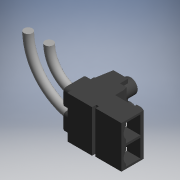
# Autodesk Inventor part: 4021832 2GD-1RR7.62-CLP-CBL
Saved by Autodesk Inventor 2017.3 (Build 213256000, 256)
## iProperties
Part Number: 4021832 2GD-1RR7.62-CLP-CBL
Material: Generic
Catalog Web Link: www.cadenas.de
Description: CMMT-plug-plug
Vendor: FESTO
Document SubType Name: Modeling
Designer: partserver
Manufacturer: FESTO
Mass: 2.92165 g
Surface Area: 28.4922 cm^2
Volume: 2.92165 cm^3
Density: 1 g/cm^3
Appearance: PSOLRGB-80-80-80
Category: PARTsolutions
Company: FESTO
Title: 4021832 2GD-1RR7.62-CLP-CBL
Author: Cadenas PARTsolutions
Comments: plug
PSOL_IDENT_0: {$CADENAS_DATA\23d-libs\festo\parts\c\cmmt\parts\cmmt_plug.prj},197 {VTYP=3D},{NB=4021832 2GD-1RR7.6
PSOL_IDENT_1: 2-CLP-CBL},{LINA=4021832 2GD-1RR7.62-CLP-CBL},{NN=CMMT-plug},{DATE=30.08.2019 14:28:39},{GEOMDATE=29
PSOL_IDENT_2: .03.2018 10:55:00},{VERSION=},{LINEID=10},{WBVAR=},{WBNUMERIC=}  {NB=4021832 2GD-1RR7.62-CLP-CBL},{L
PSOL_IDENT_3: INA=4021832 2GD-1RR7.62-CLP-CBL},{KT=DUMMY},{TNR=4021832},{TYP=2GD-1RR7.62-CLP-CBL}
NB: 4021832 2GD-1RR7.62-CLP-CBL
NN: CMMT-plug
NT: plug
NBSYN: $TNR. $TYP.
LINA: 4021832 2GD-1RR7.62-CLP-CBL
CATALOG: Festo
TNR: 4021832
TYP: 2GD-1RR7.62-CLP-CBL
SUPPLIER: FESTO
ARTICLENO: 4021832 2GD-1RR7.62-CLP-CBL
BOMINFO: 4021832 2GD-1RR7.62-CLP-CBL
CREATOR: CADENAS GmbH
Autodesk Inventor part; units mm, degrees
sketch "Sketch_1" plane through (0, 0, 0) normal (0, 0, 1) x (1, 0, 0)
  line L0 (0, 0) -> (9.3, 0)
  line L1 (9.3, 0) -> (9.3, 1.2)
  line L2 (9.3, 1.2) -> (10.2, 1.2)
  line L3 (10.2, 1.2) -> (10.2, -0.3)
  line L4 (10.2, -0.3) -> (18.85, -0.3)
  arc A0 (18.85, -0.3) -> (19.15, 0) centre (18.85, 0) ccw
  line L5 (19.15, 0) -> (19.15, 9.1)
  arc A1 (19.15, 9.1) -> (18.85, 9.4) centre (18.85, 9.1) ccw
  line L6 (18.85, 9.4) -> (17.8626, 15)
  line L7 (17.8626, 15) -> (12.6, 15)
  line L8 (12.6, 15) -> (12.6, 12.1)
  line L9 (12.6, 12.1) -> (10.2, 12.1)
  line L10 (10.2, 12.1) -> (9.83, 10.7191)
  line L11 (9.83, 10.7191) -> (9.83, 7.6)
  line L12 (9.83, 7.6) -> (3, 7.6)
  line L13 (3, 7.6) -> (3, 8.5)
  line L14 (3, 8.5) -> (1.3463, 8.5)
  line L15 (1.3463, 8.5) -> (0, 8.01)
  line L16 (0, 8.01) -> (0, 0)
  constraints: 34 end point, 4 point on circle, 2 centre point
extrude "Extrusion1" add sketch "Sketch_1" along normal mid plane 15.04
sketch "Sketch_2" plane through (13.8, 0, 0) normal (1, 0, 0) x (0, 0, -1)
  line L0 (3.81, 12.1) -> (3.81, 17.2)
  line L1 (3.81, 17.2) -> (6.11, 17.2)
  arc A0 (6.41, 16.9) -> (6.11, 17.2) centre (6.11, 16.9) ccw
  line L2 (6.41, 16.9) -> (6.41, 12.1)
  line L3 (6.41, 12.1) -> (3.81, 12.1)
  line L4 (3.81, 12.1) -> (3.81, 17.2)
  constraints: 10 end point, 2 point on circle, 1 centre point
revolve "Revolution1" add sketch "Sketch_2" angle 360 about axis through (13.8, 12.1, -3.81) along (0, -1, 0)
sketch "Sketch_3" plane through (13.8, 0, 0) normal (1, 0, 0) x (0, 0, -1)
  line L0 (-3.81, 12.1) -> (-3.81, 17.2)
  line L1 (-3.81, 17.2) -> (-1.51, 17.2)
  arc A0 (-1.21, 16.9) -> (-1.51, 17.2) centre (-1.51, 16.9) ccw
  line L2 (-1.21, 16.9) -> (-1.21, 12.1)
  line L3 (-1.21, 12.1) -> (-3.81, 12.1)
  line L4 (-3.81, 12.1) -> (-3.81, 17.2)
  constraints: 10 end point, 2 point on circle, 1 centre point
revolve "Revolution2" add sketch "Sketch_3" angle 360 about axis through (13.8, 12.1, 3.81) along (0, -1, 0)
sketch "Sketch_4" plane through (13.8, 0, 0) normal (1, 0, 0) x (0, 0, -1)
  line L0 (3.81, 13.355) -> (3.81, 17.2)
  line L1 (3.81, 17.2) -> (5.81, 17.2)
  line L2 (5.81, 17.2) -> (5.81, 13.355)
  line L3 (5.81, 13.355) -> (3.81, 13.355)
  line L4 (3.81, 13.355) -> (3.81, 17.2)
  constraints: 10 end point
revolve "Revolution3" cut sketch "Sketch_4" angle 360 about axis through (13.8, 13.355, -3.81) along (0, -1, 0)
sketch "Sketch_5" plane through (13.8, 0, 0) normal (1, 0, 0) x (0, 0, -1)
  line L0 (-3.81, 13.355) -> (-3.81, 17.2)
  line L1 (-3.81, 17.2) -> (-1.81, 17.2)
  line L2 (-1.81, 17.2) -> (-1.81, 13.355)
  line L3 (-1.81, 13.355) -> (-3.81, 13.355)
  line L4 (-3.81, 13.355) -> (-3.81, 17.2)
  constraints: 10 end point
revolve "Revolution4" cut sketch "Sketch_5" angle 360 about axis through (13.8, 13.355, 3.81) along (0, -1, 0)
sketch "Sketch_6" plane through (0, 17.2, 0) normal (0, 1, 0) x (1, 0, 0)
  line L0 (13.45, 5.6775) -> (13.45, 1.9425)
  arc A0 (13.45, 1.9425) -> (14.15, 1.9425) centre (13.8, 3.81) ccw
  line L1 (14.15, 1.9425) -> (14.15, 5.6775)
  arc A1 (14.15, 5.6775) -> (13.45, 5.6775) centre (13.8, 3.81) ccw
  constraints: 4 end point, 4 point on circle, 2 centre point
extrude "Extrusion2" cut sketch "Sketch_6" against normal blind 4.845
sketch "Sketch_7" plane through (0, 17.2, 0) normal (0, 1, 0) x (1, 0, 0)
  line L0 (13.45, -1.9425) -> (13.45, -5.6775)
  arc A0 (13.45, -5.6775) -> (14.15, -5.6775) centre (13.8, -3.81) ccw
  line L1 (14.15, -5.6775) -> (14.15, -1.9425)
  arc A1 (14.15, -1.9425) -> (13.45, -1.9425) centre (13.8, -3.81) ccw
  constraints: 4 end point, 4 point on circle, 2 centre point
extrude "Extrusion3" cut sketch "Sketch_7" against normal blind 4.845
sketch "Sketch_8" plane through (18.65, 0, 0) normal (1, 0, 0) x (0, 0, -1)
  arc A0 (-6.81, 2.2) -> (-5.81, 1.2) centre (-5.81, 2.2) ccw
  line L0 (-5.81, 1.2) -> (-1.81, 1.2)
  arc A1 (-1.81, 1.2) -> (-0.81, 2.2) centre (-1.81, 2.2) ccw
  line L1 (-0.81, 2.2) -> (-0.81, 8.4)
  arc A2 (-0.81, 8.4) -> (-1.81, 9.4) centre (-1.81, 8.4) ccw
  line L2 (-1.81, 9.4) -> (-5.81, 9.4)
  arc A3 (-5.81, 9.4) -> (-6.81, 8.4) centre (-5.81, 8.4) ccw
  line L3 (-6.81, 8.4) -> (-6.81, 2.2)
  arc A4 (-6.31, 2.2) -> (-5.81, 1.7) centre (-5.81, 2.2) ccw
  line L4 (-5.81, 1.7) -> (-1.81, 1.7)
  arc A5 (-1.81, 1.7) -> (-1.31, 2.2) centre (-1.81, 2.2) ccw
  line L5 (-1.31, 2.2) -> (-1.31, 8.4)
  arc A6 (-1.31, 8.4) -> (-1.81, 8.9) centre (-1.81, 8.4) ccw
  line L6 (-1.81, 8.9) -> (-5.81, 8.9)
  arc A7 (-5.81, 8.9) -> (-6.31, 8.4) centre (-5.81, 8.4) ccw
  line L7 (-6.31, 8.4) -> (-6.31, 2.2)
  constraints: 16 end point, 16 point on circle, 8 centre point
extrude "Extrusion4" add sketch "Sketch_8" along normal blind 3.3
sketch "Sketch_9" plane through (18.65, 0, 0) normal (1, 0, 0) x (0, 0, -1)
  arc A0 (0.81, 2.2) -> (1.81, 1.2) centre (1.81, 2.2) ccw
  line L0 (1.81, 1.2) -> (5.81, 1.2)
  arc A1 (5.81, 1.2) -> (6.81, 2.2) centre (5.81, 2.2) ccw
  line L1 (6.81, 2.2) -> (6.81, 8.4)
  arc A2 (6.81, 8.4) -> (5.81, 9.4) centre (5.81, 8.4) ccw
  line L2 (5.81, 9.4) -> (1.81, 9.4)
  arc A3 (1.81, 9.4) -> (0.81, 8.4) centre (1.81, 8.4) ccw
  line L3 (0.81, 8.4) -> (0.81, 2.2)
  arc A4 (1.31, 2.2) -> (1.81, 1.7) centre (1.81, 2.2) ccw
  line L4 (1.81, 1.7) -> (5.81, 1.7)
  arc A5 (5.81, 1.7) -> (6.31, 2.2) centre (5.81, 2.2) ccw
  line L5 (6.31, 2.2) -> (6.31, 8.4)
  arc A6 (6.31, 8.4) -> (5.81, 8.9) centre (5.81, 8.4) ccw
  line L6 (5.81, 8.9) -> (1.81, 8.9)
  arc A7 (1.81, 8.9) -> (1.31, 8.4) centre (1.81, 8.4) ccw
  line L7 (1.31, 8.4) -> (1.31, 2.2)
  constraints: 16 end point, 16 point on circle, 8 centre point
extrude "Extrusion5" add sketch "Sketch_9" along normal blind 3.3
sketch "Sketch_10" plane through (0, 0, 0) normal (1, 0, 0) x (0, 1, 0)
  line L0 (6.8, 6.82) -> (1.6, 6.82)
  line L1 (1.6, 6.82) -> (1.6, 5.8691)
  arc A0 (1.6, 5.8691) -> (1.6, 1.7509) centre (3.85, 3.81) ccw
  line L2 (1.6, 1.7509) -> (1.6, 0.4)
  line L3 (1.6, 0.4) -> (6.8, 0.4)
  line L4 (6.8, 0.4) -> (6.8, 6.82)
  constraints: 10 end point, 2 point on circle, 1 centre point
extrude "Extrusion6" cut sketch "Sketch_10" along normal blind 8.5
sketch "Sketch_11" plane through (0, 0, 0) normal (1, 0, 0) x (0, 1, 0)
  line L0 (6.8, -0.4) -> (1.6, -0.4)
  line L1 (1.6, -0.4) -> (1.6, -1.7509)
  arc A0 (1.6, -1.7509) -> (1.6, -5.8691) centre (3.85, -3.81) ccw
  line L2 (1.6, -5.8691) -> (1.6, -6.82)
  line L3 (1.6, -6.82) -> (6.8, -6.82)
  line L4 (6.8, -6.82) -> (6.8, -0.4)
  constraints: 10 end point, 2 point on circle, 1 centre point
extrude "Extrusion7" cut sketch "Sketch_11" along normal blind 8.5
sketch "Sketch_12" plane through (8.5, 0, 0) normal (1, 0, 0) x (0, 0, -1)
  line L0 (-4.31, 4.305) -> (-4.31, 3.305)
  line L1 (-4.31, 3.305) -> (-3.31, 3.305)
  line L2 (-3.31, 3.305) -> (-3.31, 4.305)
  line L3 (-3.31, 4.305) -> (-4.31, 4.305)
  constraints: 8 end point
extrude "Extrusion8" add sketch "Sketch_12" against normal blind 6.25
sketch "Sketch_13" plane through (8.5, 0, 0) normal (1, 0, 0) x (0, 0, -1)
  line L0 (3.31, 4.305) -> (3.31, 3.305)
  line L1 (3.31, 3.305) -> (4.31, 3.305)
  line L2 (4.31, 3.305) -> (4.31, 4.305)
  line L3 (4.31, 4.305) -> (3.31, 4.305)
  constraints: 8 end point
extrude "Extrusion9" add sketch "Sketch_13" against normal blind 6.25
sketch "Sketch_14" plane through (19.15, 0, 0) normal (1, 0, 0) x (0, 0, -1)
  line L0 (15, 6) -> (15, 3)
  circle A0 centre (-3.75, 4.5) radius 1.5
  constraints: 2 end point, 1 centre point
revolve "Revolution5" add sketch "Sketch_14" angle 90 about axis through (19.15, 6, -15) along (0, 1, 0)
sketch "Sketch_15" plane through (19.15, 0, 0) normal (1, 0, 0) x (0, 0, -1)
  line L0 (15, 6) -> (15, 3)
  circle A0 centre (3.75, 4.5) radius 1.5
  constraints: 2 end point, 1 centre point
revolve "Revolution6" add sketch "Sketch_15" angle 90 about axis through (19.15, 6, -15) along (0, 1, 0)
ref_plane "ANBAU_XY" through (0, 3.805, 3.81) normal (1, 0, 0) x (0, 0, -1)
ref_plane "ANBAU_YZ" through (0, 3.805, 3.81) normal (0, 0, -1) x (0, 1, 0)
ref_plane "ANBAU_ZX" through (0, 3.805, 3.81) normal (0, 1, 0) x (1, 0, 0)
body "Solid1"
